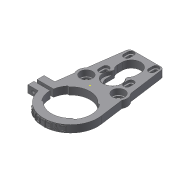
# Autodesk Inventor part: Cycl_carroZ_superior
Saved by Autodesk Inventor 2015 SP2 (Build 190223200, 223)
## iProperties
Created: 2015-05-08
Material: Genérico
Document SubType Name: Modeling
Designer: E.Beroiz
Density: 1 g/cm^3
Appearance: Valor por defecto
Description: Cycl_carroZ_superior
Author: EDU
Autodesk Inventor part; units mm, degrees
sketch "Boceto1" plane through (0, 0, 0) normal (0, 0, 1) x (1, 0, 0)
  line L0 (-5.5, 45.4273) -> (-5.5, 39.5759)
  line L1 (-2.1591, 32.4057) -> (-2.1591, 21.95)
  line L2 (14.2409, 21.95) -> (14.2409, 32.4057)
  line L3 (17.5, 40.2515) -> (17.5, 45.4273)
  line L4 (-11.5, 61.1) -> (-11.5, 56.1)
  line L5 (-7.8, 56.1) -> (-7.8, 61.1)
  line L6 (27.5298, 60.9274) -> (33.5477, 17.1)
  line L7 (35.334, 4.0901) -> (39.4073, -25.5751)
  line L8 (-26.7015, -37.5504) -> (-39.593, -37.5504)
  line L9 (-39.593, -37.5504) -> (-39.593, -30.0504)
  line L10 (-39.593, -30.0504) -> (-19.5686, -30.0504)
  line L11 (-13.9951, -46.0504) -> (-11.6451, -46.0504)
  line L12 (23.8386, -46.0504) -> (26.1886, -46.0504)
  line L13 (26.01, -14.0504) -> (23.66, -14.0504)
  line L14 (-11.4665, -14.0504) -> (-13.8165, -14.0504)
  line L15 (-19.2523, -26.1608) -> (-39.5688, -26.1608)
  line L16 (-39.5688, -26.1608) -> (-39.5688, -17.572)
  line L17 (-39.5688, -17.572) -> (-26.2755, -17.572)
  line L18 (-26.2755, -17.572) -> (-23.3041, 4.0684)
  line L19 (-21.5178, 17.0782) -> (-15.5579, 60.4837)
  line L20 (-11.0096, 64.4501) -> (23.4904, 64.4501)
  circle A0 centre (-13.9561, 10.0982) radius 6
  circle A1 centre (26.0439, 10.0982) radius 6
  arc A2 (-26.7015, -37.5504) -> (39.4073, -25.5751) centre (6.0968, -30.1489) ccw
  arc A3 (35.334, 4.0901) -> (33.5477, 17.1) centre (25.8546, 9.4161) ccw
  arc A4 (-21.5178, 17.0782) -> (-23.3041, 4.0684) centre (-13.9561, 9.4124) ccw
  arc A5 (17.5, 45.4273) -> (-5.5, 45.4273) centre (6, 45.4273) ccw
  arc A6 (-5.5, 39.5759) -> (-2.1591, 32.4057) centre (3.8649, 39.5759) ccw
  arc A7 (14.2409, 32.4057) -> (17.5, 40.2515) centre (6.4267, 40.2515) ccw
  arc A8 (-7.8, 61.1) -> (-11.5, 61.1) centre (-9.65, 61.1) ccw
  arc A9 (-11.5, 56.1) -> (-7.8, 56.1) centre (-9.65, 56.1) ccw
  arc A10 (-11.0096, 64.4501) -> (-15.5579, 60.4837) centre (-11.0096, 59.8592) ccw
  arc A11 (27.5298, 60.9274) -> (23.4904, 64.4501) centre (23.4904, 60.3728) ccw
  arc A12 (-2.1591, 21.95) -> (14.2409, 21.95) centre (6.0409, 21.95) ccw
  circle A13 centre (6.0968, -30.1489) radius 23.825
  arc A14 (-13.8165, -14.0504) -> (-13.9951, -46.0504) centre (5.8673, -30.1608) ccw
  arc A15 (26.1886, -46.0504) -> (26.01, -14.0504) centre (6.3262, -30.1608) ccw
  point P0 (0, 0)
  point P1 (0, 0)
  point P2 (6, 56.9273)
  dimension "d1" = 0
  dimension "d14" = 12
  dimension "d15" = 12
  dimension "d16" = 40
  dimension "d46" = 1.85
  dimension "d47" = 1.85
  dimension "d51" = 5
  dimension "d52" = 5
  dimension "d54" = 34.5
  dimension "d72" = 8.2
  dimension "d74" = 47.65
  dimension "d75" = 2.35
  dimension "d76" = 2.35
  dimension "d77" = 2.35
  dimension "d78" = 2.35
  dimension "d79" = 25.4361
  dimension "d80" = 25.4361
  dimension "d95" = 40.2471
  constraints: 42 end point, 33 point on circle, 16 centre point, 15 tangent, 3 vertical alignment, 1 coincident, 1 horizontal alignment
  measures "d14" diameter of A0
  measures "d15" diameter of A1
  measures "d16" distance of A0.centre A1.centre
  measures "d46" radius of A8
  measures "d47" radius of A9
  measures "d51" distance of L5.start L5.end
  measures "d52" distance of L4.start L4.end
  measures "d54" distance of L20.start L20.end
  measures "d72" radius of A12
  measures "d74" diameter of A13
  measures "d75" distance of L14.start L14.end
  measures "d76" distance of L11.start L11.end
  measures "d77" distance of L13.start L13.end
  measures "d78" distance of L12.start L12.end
  measures "d79" radius of A14
  measures "d80" radius of A15
  measures "d95" vertical distance of A13.centre A1.centre
extrude "Extrusión1" add sketch "Boceto1" along normal blind 9 contours A8 L5 A9 L4 | L6 A3 L7 A2 L8 L9 L10 A14 L11 A13 L12 A15 L13 L14 L15 L16 L17 L18 A4 L19 A10 L20 A11 | A0 | A1
sketch "Boceto2" plane through (0, 0, 9) normal (0, 0, 1) x (1, 0, 0)
  line L0 (17.5, 45.4273) -> (17.5, 40.2515) projected
  line L1 (14.2409, 32.4057) -> (14.2409, 21.95) projected
  line L2 (-2.1591, 21.95) -> (-2.1591, 32.4057) projected
  line L3 (-5.5, 39.5759) -> (-5.5, 45.4273) projected
  line L4 (23.4904, 64.4501) -> (-11.0096, 64.4501) projected
  line L5 (-15.5579, 60.4837) -> (-21.5178, 17.0782) projected
  line L6 (-23.3041, 4.0684) -> (-26.2755, -17.572) projected
  line L7 (-26.2755, -17.572) -> (-39.5688, -17.572) projected
  line L8 (-39.5688, -17.572) -> (-39.5688, -26.1608) projected
  line L9 (-39.5688, -26.1608) -> (-19.2523, -26.1608) projected
  line L10 (-13.8165, -14.0504) -> (-11.4665, -14.0504) projected
  line L11 (23.66, -14.0504) -> (26.01, -14.0504) projected
  line L12 (26.1886, -46.0504) -> (23.8386, -46.0504) projected
  line L13 (-11.6451, -46.0504) -> (-13.9951, -46.0504) projected
  line L14 (-19.5686, -30.0504) -> (-39.593, -30.0504) projected
  line L15 (-39.593, -30.0504) -> (-39.593, -37.5504) projected
  line L16 (-39.593, -37.5504) -> (-26.7015, -37.5504) projected
  line L17 (39.4073, -25.5751) -> (35.334, 4.0901) projected
  line L18 (33.5477, 17.1) -> (27.5298, 60.9274) projected
  circle A0 centre (-13.9913, 9.45) radius 7.725
  circle A1 centre (26.0087, 9.45) radius 7.725
  arc A2 (-26.7015, -37.5504) -> (39.4073, -25.5751) centre (6.0968, -30.1489) ccw projected
  arc A3 (-21.5178, 17.0782) -> (-23.3041, 4.0684) centre (-13.9561, 9.4124) ccw projected
  arc A4 (35.334, 4.0901) -> (33.5477, 17.1) centre (25.8546, 9.4161) ccw projected
  arc A5 (17.5, 45.4273) -> (-5.5, 45.4273) centre (6, 45.4273) ccw projected
  arc A6 (14.2409, 32.4057) -> (17.5, 40.2515) centre (6.4267, 40.2515) ccw projected
  arc A7 (-5.5, 39.5759) -> (-2.1591, 32.4057) centre (3.8649, 39.5759) ccw projected
  arc A8 (27.5298, 60.9274) -> (23.4904, 64.4501) centre (23.4904, 60.3728) ccw projected
  arc A9 (-11.0096, 64.4501) -> (-15.5579, 60.4837) centre (-11.0096, 59.8592) ccw projected
  arc A10 (-2.1591, 21.95) -> (14.2409, 21.95) centre (6.0409, 21.95) ccw projected
  arc A11 (23.66, -14.0504) -> (-11.4665, -14.0504) centre (6.0968, -30.1489) ccw projected
  arc A12 (-11.6451, -46.0504) -> (23.8386, -46.0504) centre (6.0968, -30.1489) ccw projected
  arc A13 (-13.8165, -14.0504) -> (-19.2523, -26.1608) centre (5.8673, -30.1608) ccw projected
  arc A14 (-19.5686, -30.0504) -> (-13.9951, -46.0504) centre (5.8673, -30.1608) ccw projected
  arc A15 (26.1886, -46.0504) -> (26.01, -14.0504) centre (6.3262, -30.1608) ccw projected
  point P0 (0, 0)
  dimension "d1" = 0
  dimension "d2" = 15.45
  dimension "d3" = 15.45
  dimension "d19" = 40
  constraints: 2 centre point, 1 horizontal alignment
  measures "d2" diameter of A0
  measures "d3" diameter of A1
  measures "d19" distance of A1.centre A0.centre
extrude "Extrusión4" cut sketch "Boceto2" against normal blind 10 contours A0 | A1
sketch "Boceto5" plane through (0, 0, 0) normal (0, 0, -1) x (-1, 0, 0)
  circle A0 centre (13.9913, 9.45) radius 7.725 projected
  circle A1 centre (-26.0087, 9.45) radius 7.725 projected
  circle A2 centre (13.9913, 9.45) radius 6
  circle A3 centre (-26.0087, 9.45) radius 6
  point P0 (0, 0)
  dimension "d22" = 12
  dimension "d23" = 12
  constraints: 2 centre point, 2 coincident
  measures "d22" diameter of A2
  measures "d23" diameter of A3
extrude "Extrusión5" add sketch "Boceto5" against normal blind 2
sketch "Boceto7" plane through (0, 0, 9) normal (0, 0, 1) x (1, 0, 0)
  circle A0 centre (-13.9913, 9.45) radius 7.725 projected
  circle A1 centre (26.0087, 9.45) radius 7.725 projected
  line L0 (17.5, 45.4273) -> (17.5, 40.2515) projected
  line L1 (14.2409, 32.4057) -> (14.2409, 21.95) projected
  line L2 (-2.1591, 21.95) -> (-2.1591, 32.4057) projected
  line L3 (-5.5, 39.5759) -> (-5.5, 45.4273) projected
  line L4 (-15.5579, 60.4837) -> (-21.5178, 17.0782) projected
  line L5 (-23.3041, 4.0684) -> (-26.2755, -17.572) projected
  line L6 (-26.2755, -17.572) -> (-39.5688, -17.572) projected
  line L7 (-39.5688, -17.572) -> (-39.5688, -26.1608) projected
  line L8 (-39.5688, -26.1608) -> (-19.2523, -26.1608) projected
  line L9 (-13.8165, -14.0504) -> (-11.4665, -14.0504) projected
  line L10 (23.66, -14.0504) -> (26.01, -14.0504) projected
  line L11 (26.1886, -46.0504) -> (23.8386, -46.0504) projected
  line L12 (-11.6451, -46.0504) -> (-13.9951, -46.0504) projected
  line L13 (-19.5686, -30.0504) -> (-39.593, -30.0504) projected
  line L14 (-39.593, -30.0504) -> (-39.593, -37.5504) projected
  line L15 (-39.593, -37.5504) -> (-26.7015, -37.5504) projected
  line L16 (39.4073, -25.5751) -> (35.334, 4.0901) projected
  line L17 (33.5477, 17.1) -> (27.5298, 60.9274) projected
  line L18 (23.4904, 64.4501) -> (-11.0096, 64.4501) projected
  circle A2 centre (6, -30) radius 24
  arc A3 (-26.7015, -37.5504) -> (39.4073, -25.5751) centre (6.0968, -30.1489) ccw projected
  arc A4 (-21.5178, 17.0782) -> (-23.3041, 4.0684) centre (-13.9561, 9.4124) ccw projected
  arc A5 (35.334, 4.0901) -> (33.5477, 17.1) centre (25.8546, 9.4161) ccw projected
  arc A6 (17.5, 45.4273) -> (-5.5, 45.4273) centre (6, 45.4273) ccw projected
  arc A7 (14.2409, 32.4057) -> (17.5, 40.2515) centre (6.4267, 40.2515) ccw projected
  arc A8 (-5.5, 39.5759) -> (-2.1591, 32.4057) centre (3.8649, 39.5759) ccw projected
  arc A9 (27.5298, 60.9274) -> (23.4904, 64.4501) centre (23.4904, 60.3728) ccw projected
  arc A10 (-11.0096, 64.4501) -> (-15.5579, 60.4837) centre (-11.0096, 59.8592) ccw projected
  arc A11 (-2.1591, 21.95) -> (14.2409, 21.95) centre (6.0409, 21.95) ccw projected
  arc A12 (23.66, -14.0504) -> (-11.4665, -14.0504) centre (6.0968, -30.1489) ccw projected
  arc A13 (-11.6451, -46.0504) -> (23.8386, -46.0504) centre (6.0968, -30.1489) ccw projected
  arc A14 (-13.8165, -14.0504) -> (-19.2523, -26.1608) centre (5.8673, -30.1608) ccw projected
  arc A15 (-19.5686, -30.0504) -> (-13.9951, -46.0504) centre (5.8673, -30.1608) ccw projected
  arc A16 (26.1886, -46.0504) -> (26.01, -14.0504) centre (6.3262, -30.1608) ccw projected
  point P0 (0, 0)
  dimension "d1" = 0
  dimension "d26" = 48
  dimension "d27" = 30
  dimension "d28" = 6
  constraints: 1 centre point
  measures "d26" diameter of A2
  measures "d27" vertical distance of A2.centre point (0, 0)
  measures "d28" horizontal distance of A2.centre point (0, 0)
extrude "Extrusión6" cut sketch "Boceto7" against normal through all contours A2 L10 A12 L9 | L9 A12 L10 A2 L11 A13 L12 | L12 A13 A2 | A2 A13 | A2 A13 L11
sketch "Boceto10" plane through (-39.593, -37.5504, 0) normal (0, -1, 0) x (1, 0, 0)
  line L0 (13.3176, 0) -> (0.0242, 0) projected
  line L1 (0, 0) -> (0, 9) projected
  point P0 (39.593, 0)
  point P1 (6.6709, 4.5)
  point P2 (6.6709, 0)
  point P3 (0, 4.5)
  constraints: 1 horizontal alignment, 1 midpoint, 1 vertical alignment, 2 other
hole "Agujero1" at (-32.9222, -37.5504, 4.5) direction (0, 1, 0) diameter 3.75 end through all
sketch "Boceto11" plane through (-39.5688, -17.572, 0) normal (0, 1, 0) x (1, 0, 0)
  circle A0 centre (6.6467, -4.5) radius 1.875 projected
  line L0 (8.4466, -1.3825) -> (10.2464, -4.5)
  line L1 (10.2464, -4.5) -> (8.4466, -7.6175)
  line L2 (8.4466, -7.6175) -> (4.8468, -7.6175)
  line L3 (4.8468, -7.6175) -> (3.0469, -4.5)
  line L4 (3.0469, -4.5) -> (4.8468, -1.3825)
  line L5 (4.8468, -1.3825) -> (8.4466, -1.3825)
  point P0 (39.5688, 0)
  dimension "d43" = 6.235
  constraints: 12 end point, 1 coincident, 1 horizontal, 13 other
  measures "d43" distance between parallel lines of L2 L5
extrude "Extrusión8" cut sketch "Boceto11" against normal blind 2.8
sketch "Boceto12" plane through (0, 0, 9) normal (0, 0, 1) x (1, 0, 0)
  line L0 (23.4904, 64.4501) -> (-11.0096, 64.4501) projected
  line L1 (-11.1096, 59.9501) -> (-11.1096, 54.9501)
  arc A0 (-11.1096, 54.9501) -> (-7.4096, 54.9501) centre (-9.2596, 54.9501) ccw
  line L2 (-7.4096, 54.9501) -> (-7.4096, 59.9501)
  arc A1 (-7.4096, 59.9501) -> (-11.1096, 59.9501) centre (-9.2596, 59.9501) ccw
  line L3 (-9.2596, 59.9501) -> (6.2404, 59.9501) construction
  point P0 (0, 0)
  point P1 (6.2404, 64.4501)
  dimension "d59" = 5
  dimension "d60" = 5
  dimension "d61" = 1.85
  dimension "d62" = 15.5
  dimension "d63" = 4.5
  constraints: 6 end point, 4 point on circle, 3 tangent, 2 centre point, 2 vertical, 1 horizontal, 1 midpoint, 1 vertical alignment
  measures "d59" distance of L1.start L1.end
  measures "d60" distance of L2.start L2.end
  measures "d61" radius of A1
  measures "d62" distance of L3.start L3.end
  measures "d63" distance from line of L0 L3.start
extrude "Extrusión10" cut sketch "Boceto12" against normal through all
pattern_linear "Patrón rectangular1" count 2 spacing 31 along (0, -1, 0) count 2 spacing 31 along (1, 0, 0) of "Extrusión10"
sketch "Boceto13" plane through (0, 0, 9) normal (0, 0, 1) x (1, 0, 0)
  arc A0 (23.5904, 28.9501) -> (19.8904, 28.9501) centre (21.7404, 28.9501) ccw projected
  line L0 (23.5904, 28.9501) -> (23.5904, 23.9501) projected
  arc A1 (19.8904, 23.9501) -> (23.5904, 23.9501) centre (21.7404, 23.9501) ccw projected
  line L1 (19.8904, 23.9501) -> (19.8904, 28.9501) projected
  arc A2 (23.5904, 59.9501) -> (19.8904, 59.9501) centre (21.7404, 59.9501) ccw projected
  line L2 (23.5904, 59.9501) -> (23.5904, 54.9501) projected
  arc A3 (19.8904, 54.9501) -> (23.5904, 54.9501) centre (21.7404, 54.9501) ccw projected
  line L3 (19.8904, 54.9501) -> (19.8904, 59.9501) projected
  arc A4 (-7.4096, 28.9501) -> (-11.1096, 28.9501) centre (-9.2596, 28.9501) ccw projected
  line L4 (-7.4096, 28.9501) -> (-7.4096, 23.9501) projected
  arc A5 (-11.1096, 23.9501) -> (-7.4096, 23.9501) centre (-9.2596, 23.9501) ccw projected
  line L5 (-11.1096, 23.9501) -> (-11.1096, 28.9501) projected
  arc A6 (-11.1096, 54.9501) -> (-7.4096, 54.9501) centre (-9.2596, 54.9501) ccw projected
  line L6 (-11.1096, 54.9501) -> (-11.1096, 59.9501) projected
  arc A7 (-7.4096, 59.9501) -> (-11.1096, 59.9501) centre (-9.2596, 59.9501) ccw projected
  line L7 (-7.4096, 59.9501) -> (-7.4096, 54.9501) projected
  arc A8 (-11.8433, -46.0504) -> (15.4729, -52.0514) centre (6, -30) ccw projected
  line L8 (-11.8433, -46.0504) -> (-13.9951, -46.0504) projected
  arc A9 (-19.5686, -30.0504) -> (-13.9951, -46.0504) centre (5.8673, -30.1608) ccw projected
  line L9 (-19.5686, -30.0504) -> (-39.593, -30.0504) projected
  line L10 (-39.593, -30.0504) -> (-39.593, -37.5504) projected
  line L11 (-39.593, -37.5504) -> (-26.7015, -37.5504) projected
  arc A10 (-26.7015, -37.5504) -> (39.4073, -25.5751) centre (6.0968, -30.1489) ccw projected
  line L12 (39.4073, -25.5751) -> (35.334, 4.0901) projected
  arc A11 (35.334, 4.0901) -> (33.5477, 17.1) centre (25.8546, 9.4161) ccw projected
  line L13 (33.5477, 17.1) -> (27.5298, 60.9274) projected
  arc A12 (27.5298, 60.9274) -> (23.4904, 64.4501) centre (23.4904, 60.3728) ccw projected
  line L14 (23.4904, 64.4501) -> (-11.0096, 64.4501) projected
  arc A13 (-11.0096, 64.4501) -> (-15.5579, 60.4837) centre (-11.0096, 59.8592) ccw projected
  line L15 (-15.5579, 60.4837) -> (-21.5178, 17.0782) projected
  arc A14 (-21.5178, 17.0782) -> (-23.3041, 4.0684) centre (-13.9561, 9.4124) ccw projected
  line L16 (-23.3041, 4.0684) -> (-26.2755, -17.572) projected
  line L17 (-26.2755, -17.572) -> (-39.5688, -17.572) projected
  line L18 (-39.5688, -17.572) -> (-39.5688, -26.1608) projected
  line L19 (-39.5688, -26.1608) -> (-19.2523, -26.1608) projected
  arc A15 (-13.8165, -14.0504) -> (-19.2523, -26.1608) centre (5.8673, -30.1608) ccw projected
  line L20 (-13.8165, -14.0504) -> (-11.9335, -14.0504) projected
  arc A16 (23.9335, -14.0504) -> (-11.9335, -14.0504) centre (6, -30) ccw projected
  line L21 (23.9335, -14.0504) -> (26.01, -14.0504) projected
  arc A17 (26.1886, -46.0504) -> (26.01, -14.0504) centre (6.3262, -30.1608) ccw projected
  line L22 (26.1886, -46.0504) -> (23.8433, -46.0504) projected
  arc A18 (22.2999, -47.6157) -> (23.8433, -46.0504) centre (6, -30) ccw projected
  arc A19 (15.4729, -52.0514) -> (22.2999, -47.6157) centre (6.0968, -30.1489) ccw projected
  circle A20 centre (-13.9913, 9.45) radius 7.725 projected
  circle A21 centre (26.0087, 9.45) radius 7.725 projected
  arc A22 (17.5, 45.4273) -> (-5.5, 45.4273) centre (6, 45.4273) ccw projected
  line L23 (17.5, 45.4273) -> (17.5, 40.2515) projected
  arc A23 (14.2409, 32.4057) -> (17.5, 40.2515) centre (6.4267, 40.2515) ccw projected
  line L24 (14.2409, 32.4057) -> (14.2409, 21.95) projected
  arc A24 (-2.1591, 21.95) -> (14.2409, 21.95) centre (6.0409, 21.95) ccw projected
  line L25 (-2.1591, 21.95) -> (-2.1591, 32.4057) projected
  arc A25 (-5.5, 39.5759) -> (-2.1591, 32.4057) centre (3.8649, 39.5759) ccw projected
  line L26 (-5.5, 39.5759) -> (-5.5, 45.4273) projected
  line L27 (-13.1096, 59.9501) -> (-13.1096, 54.9501)
  arc A26 (-13.1096, 54.9501) -> (-5.4096, 54.9501) centre (-9.2596, 54.9501) ccw
  line L28 (-5.4096, 54.9501) -> (-5.4096, 59.9501)
  arc A27 (-5.4096, 59.9501) -> (-13.1096, 59.9501) centre (-9.2596, 59.9501) ccw
  arc A28 (25.5904, 59.9501) -> (17.8904, 59.9501) centre (21.7404, 59.9501) ccw
  line L29 (25.5904, 59.9501) -> (25.5904, 54.9501)
  arc A29 (17.8904, 54.9501) -> (25.5904, 54.9501) centre (21.7404, 54.9501) ccw
  line L30 (17.8904, 54.9501) -> (17.8904, 59.9501)
  arc A30 (25.5904, 28.9501) -> (17.8904, 28.9501) centre (21.7404, 28.9501) ccw
  line L31 (25.5904, 28.9501) -> (25.5904, 23.9501)
  arc A31 (17.8904, 23.9501) -> (25.5904, 23.9501) centre (21.7404, 23.9501) ccw
  line L32 (17.8904, 23.9501) -> (17.8904, 28.9501)
  arc A32 (-5.4096, 28.9501) -> (-13.1096, 28.9501) centre (-9.2596, 28.9501) ccw
  line L33 (-5.4096, 28.9501) -> (-5.4096, 23.9501)
  arc A33 (-13.1096, 23.9501) -> (-5.4096, 23.9501) centre (-9.2596, 23.9501) ccw
  line L34 (-13.1096, 23.9501) -> (-13.1096, 28.9501)
  point P0 (0, 0)
  dimension "d1" = 0
  dimension "d81" = 2
  dimension "d82" = 2
  dimension "d83" = 2
  dimension "d84" = 2
  constraints: 16 end point, 16 point on circle, 8 centre point, 12 other
  measures "d81" radial gap between concentric circles of A7 A27
  measures "d82" distance between parallel lines of L3 L30
  measures "d83" distance between parallel lines of L1 L32
  measures "d84" distance between parallel lines of L5 L34
extrude "Extrusión11" cut sketch "Boceto13" against normal blind 2.8 contours A27 L28 A26 L27 | L29 A29 L30 A28 | L31 A31 L32 A30 | L33 A33 L34 A32
sketch "Boceto15" plane through (0, 0, 9) normal (0, 0, 1) x (1, 0, 0)
  point P0 (0, 0)
sketch "Boceto16" plane through (0, 0, 9) normal (0, 0, 1) x (1, 0, 0)
  arc A0 (-2.1591, 21.95) -> (14.2409, 21.95) centre (6.0409, 21.95) ccw projected
  circle A1 centre (6.0409, 21.95) radius 11.25
  point P0 (0, 0)
  dimension "d89" = 22.5
  constraints: 1 centre point, 1 coincident
  measures "d89" diameter of A1
extrude "Extrusión12" cut sketch "Boceto16" against normal blind 4.5
ref_plane "Plano de trabajo1" through (6.0164, 217.6083, 0) normal (-1, 0, 0) x (0, 0, 1)
chamfer "Chaflán1" distance 0.5 angle 30 1 edges at (6.0409, 10.7, 9)
ref_plane "Plano de trabajo6" through (6.0968, -63.772, 0) normal (0, -1, 0) x (1, 0, 0)
sketch "Boceto27" plane through (6.0968, -63.772, 0) normal (0, -1, 0) x (1, 0, 0)
  line L0 (25.7615, 0.4873) -> (-25.8733, 0.4873) construction
  line L1 (-25.8733, 0.4873) -> (-25.8733, 8.5127) construction
  line L2 (-25.8733, 8.5127) -> (25.7615, 8.5127) construction
  line L3 (25.7615, 8.5127) -> (25.7615, 0.4873) construction
  line L4 (-32.7983, 0) -> (-32.7983, 9) projected
  line L5 (-11.3059, 8.7113) -> (11.1941, 8.7113) projected
  line L6 (17.0356, 2.1311) -> (21.8588, 2.1311)
  spline S0 degree 2 poles (21.8588, 2.1311) (21.9136, 2.1311) (21.9136, 2.2043) knots 0 0 0 1 1 1
  line L7 (21.9136, 2.2043) -> (21.9136, 6.8079)
  spline S1 degree 2 poles (21.9136, 6.8079) (21.9136, 6.8811) (21.8588, 6.8811) knots 0 0 0 1 1 1
  line L8 (21.8588, 6.8811) -> (17.0356, 6.8811)
  line L9 (17.0356, 6.8811) -> (17.0356, 8.253)
  line L10 (17.0356, 8.253) -> (21.8588, 8.253)
  spline S2 degree 2 poles (21.8588, 8.253) (22.3405, 8.253) (23.0173, 7.4116) (23.0173, 6.8079) knots 0 0 0 1 2 2 2
  line L11 (23.0173, 6.8079) -> (23.0173, 2.2043)
  spline S3 degree 2 poles (23.0173, 2.2043) (23.0173, 1.6006) (22.3405, 0.753) (21.8588, 0.753) knots 0 0 0 1 2 2 2
  line L12 (21.8588, 0.753) -> (17.0356, 0.753)
  line L13 (17.0356, 0.753) -> (17.0356, 2.1311)
  line L14 (11.1697, 0.753) -> (9.8588, 0.753)
  line L15 (9.8588, 0.753) -> (12.627, 5.4543)
  line L16 (12.627, 5.4543) -> (12.627, 8.253)
  line L17 (12.627, 8.253) -> (13.7246, 8.253)
  line L18 (13.7246, 8.253) -> (13.7246, 5.4543)
  line L19 (13.7246, 5.4543) -> (16.499, 0.753)
  line L20 (16.499, 0.753) -> (15.188, 0.753)
  line L21 (15.188, 0.753) -> (13.1758, 3.9421)
  line L22 (13.1758, 3.9421) -> (11.1697, 0.753)
  line L23 (3.4868, 2.1311) -> (8.31, 2.1311)
  spline S4 degree 2 poles (8.31, 2.1311) (8.3649, 2.1311) (8.3649, 2.2043) knots 0 0 0 1 1 1
  line L24 (8.3649, 2.2043) -> (8.3649, 6.8079)
  spline S5 degree 2 poles (8.3649, 6.8079) (8.3649, 6.8811) (8.31, 6.8811) knots 0 0 0 1 1 1
  line L25 (8.31, 6.8811) -> (3.4868, 6.8811)
  line L26 (3.4868, 6.8811) -> (3.4868, 8.253)
  line L27 (3.4868, 8.253) -> (8.31, 8.253)
  spline S6 degree 2 poles (8.31, 8.253) (8.7917, 8.253) (9.4685, 7.4116) (9.4685, 6.8079) knots 0 0 0 1 2 2 2
  line L28 (9.4685, 6.8079) -> (9.4685, 2.2043)
  spline S7 degree 2 poles (9.4685, 2.2043) (9.4685, 1.6006) (8.7917, 0.753) (8.31, 0.753) knots 0 0 0 1 2 2 2
  line L29 (8.31, 0.753) -> (3.4868, 0.753)
  line L30 (3.4868, 0.753) -> (3.4868, 2.1311)
  line L31 (2.6149, 8.253) -> (2.6149, 0.747)
  line L32 (2.6149, 0.747) -> (1.5173, 0.747)
  line L33 (1.5173, 0.747) -> (1.5173, 6.8811)
  line L34 (1.5173, 6.8811) -> (-3.379, 6.8811)
  line L35 (-3.379, 6.8811) -> (-3.379, 8.253)
  line L36 (-3.379, 8.253) -> (2.6149, 8.253)
  line L37 (-5.001, 0.753) -> (-8.6839, 0.753)
  spline S8 degree 2 poles (-8.6839, 0.753) (-9.1595, 0.753) (-9.8425, 1.6006) (-9.8425, 2.2043) knots 0 0 0 1 2 2 2
  line L38 (-9.8425, 2.2043) -> (-9.8425, 6.8079)
  spline S9 degree 2 poles (-9.8425, 6.8079) (-9.8425, 7.4116) (-9.1595, 8.253) (-8.6839, 8.253) knots 0 0 0 1 2 2 2
  line L39 (-8.6839, 8.253) -> (-5.001, 8.253)
  spline S10 degree 2 poles (-5.001, 8.253) (-4.5193, 8.253) (-3.8486, 7.4116) (-3.8486, 6.8079) knots 0 0 0 1 2 2 2
  line L40 (-3.8486, 6.8079) -> (-3.8486, 2.2043)
  spline S11 degree 2 poles (-3.8486, 2.2043) (-3.8486, 1.6006) (-4.5193, 0.753) (-5.001, 0.753) knots 0 0 0 1 2 2 2
  line L41 (-5.001, 6.8811) -> (-8.6839, 6.8811)
  spline S12 degree 2 poles (-8.6839, 6.8811) (-8.7327, 6.8811) (-8.7327, 6.8079) knots 0 0 0 1 1 1
  line L42 (-8.7327, 6.8079) -> (-8.7327, 2.2043)
  spline S13 degree 2 poles (-8.7327, 2.2043) (-8.7327, 2.1311) (-8.6839, 2.1311) knots 0 0 0 1 1 1
  line L43 (-8.6839, 2.1311) -> (-5.001, 2.1311)
  spline S14 degree 2 poles (-5.001, 2.1311) (-4.9461, 2.1311) (-4.9461, 2.2043) knots 0 0 0 1 1 1
  line L44 (-4.9461, 2.2043) -> (-4.9461, 6.8079)
  spline S15 degree 2 poles (-4.9461, 6.8079) (-4.9461, 6.8811) (-5.001, 6.8811) knots 0 0 0 1 1 1
  line L45 (-15.6412, 6.253) -> (-15.6412, 0.753)
  line L46 (-15.6412, 0.753) -> (-16.7449, 0.753)
  line L47 (-16.7449, 0.753) -> (-16.7449, 8.253)
  line L48 (-16.7449, 8.253) -> (-15.5498, 8.253)
  line L49 (-15.5498, 8.253) -> (-11.8547, 2.753)
  line L50 (-11.8547, 2.753) -> (-11.8547, 8.253)
  line L51 (-11.8547, 8.253) -> (-10.751, 8.253)
  line L52 (-10.751, 8.253) -> (-10.751, 0.753)
  line L53 (-10.751, 0.753) -> (-11.9522, 0.753)
  line L54 (-11.9522, 0.753) -> (-15.6412, 6.253)
  line L55 (-23.2083, 0.753) -> (-23.2083, 2.1311)
  line L56 (-23.2083, 2.1311) -> (-18.8059, 2.1311)
  line L57 (-18.8059, 2.1311) -> (-18.8059, 3.814)
  line L58 (-18.8059, 3.814) -> (-22.3486, 3.814)
  line L59 (-22.3486, 3.814) -> (-22.3486, 5.1921)
  line L60 (-22.3486, 5.1921) -> (-18.8059, 5.1921)
  line L61 (-18.8059, 5.1921) -> (-18.8059, 6.8811)
  line L62 (-18.8059, 6.8811) -> (-23.2083, 6.8811)
  line L63 (-23.2083, 6.8811) -> (-23.2083, 8.253)
  line L64 (-23.2083, 8.253) -> (-17.6961, 8.253)
  line L65 (-17.6961, 8.253) -> (-17.6961, 0.753)
  line L66 (-17.6961, 0.753) -> (-23.2083, 0.753)
  point P0 (-0.0559, 8.5127)
  point P1 (8.1441, 8.7113)
  point P2 (-8.2559, 8.7113)
  point P3 (-32.7983, 4.5)
  point P4 (-25.8733, 4.5)
  point P5 (-0.0559, 0.4873)
  point P6 (-0.0559, 8.7113)
  constraints: 4 midpoint, 1 horizontal alignment, 1 vertical alignment, 2 other
emboss "Repujado2" sketch "Boceto27" operation add depth 0.9 direction (0, 1, 0) wrap yes faces at (39.1946, -36.0688, 6)
